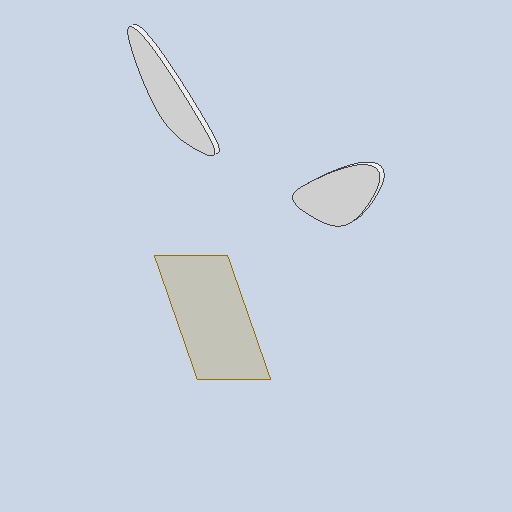
# Autodesk Inventor part: втавки в уши
Saved by Autodesk Inventor 2024.2 (Build 282272000, 272)
## iProperties
Created: 2026-04-13
Part Number: втавки в уши
Material: Типовые
Document SubType Name: Modeling
Designer: katya_notebook
Density: 1 g/cm^3
Appearance: Белый
Author: katya_notebook
Autodesk Inventor part; units mm, degrees
ref_plane "YZ Plane" through (0, 0, 0) normal (1, 0, 0) x (0, 1, 0)
ref_plane "XZ Plane" through (0, 0, 0) normal (0, 1, 0) x (-1, 0, 0)
ref_plane "XY Plane" through (0, 0, 0) normal (0, 0, 1) x (1, 0, 0)
ref_plane "РабПлоскость1" through (35.0491, -167.4778, 0) normal (0, 0, 1) x (-0.4483757, 0.8938452, 0)
sketch "Эскиз1" plane through (35.0491, -167.4778, 0) normal (0, 0, 1) x (-0.4483757, 0.8938452, 0)
  spline S0 degree 3 poles (119.1304, -59.9769) (121.6559, -53.204) (124.3274, -47.3227) (129.9976, -38.042) (132.8145, -34.5593) (139.864, -28.2576) (144.2541, -25.75) (161.0383, -19.7449) (176.2169, -18.9451) (191.3353, -18.7692) (197.9842, -18.9943) (204.6873, -20.2717) (206.5014, -20.7653) (208.7394, -21.856) (209.4736, -22.3119) (210.4771, -23.27) (210.8203, -23.7079) (211.3082, -24.6937) (211.4431, -25.2098) (211.5165, -26.4335) (211.3928, -27.1121) (210.789, -28.8946) (210.0931, -29.9834) (207.1495, -33.7221) (203.6117, -36.415) (190.7312, -44.8629) (177.0786, -50.9399) (157.9772, -58.7745) (140.9066, -65.3521) (129.32, -68.3562) (126.8697, -68.8535) (123.8804, -68.9432) (122.9917, -68.8784) (121.6982, -68.5374) (121.2096, -68.337) (120.3608, -67.7605) (120.0208, -67.412) (119.3919, -66.448) (119.1764, -65.822) (118.7753, -63.8427) (118.8182, -62.121) (119.1304, -59.9769) knots -19.535718 -19.535718 -19.535718 -19.535718 -18.521729 -18.521729 -17.645169 -17.645169 -16.585337 -16.585337 -14.272905 -14.272905 -12.64955 -12.64955 -12.036111 -12.036111 -11.729258 -11.729258 -11.523538 -11.523538 -11.322846 -11.322846 -11.070518 -11.070518 -10.627583 -10.627583 -9.313537 -9.313537 -5.689602 -5.689602 -2.653594 -2.653594 -1.828822 -1.828822 -1.444244 -1.444244 -1.194814 -1.194814 -0.958616 -0.958616 -0.650005 -0.650005 0 0 0 0 projected
  spline S1 degree 3 poles (81.1608, -135.4055) (82.6694, -133.905) (84.0051, -132.8572) (85.7594, -132.0121) (86.3344, -131.8139) (87.4209, -131.6843) (87.9054, -131.7157) (88.9368, -132.0027) (89.437, -132.2802) (90.5464, -133.1347) (91.1457, -133.8196) (92.6734, -135.997) (93.6462, -137.8968) (98.3538, -149.2241) (103.4784, -167.8703) (108.7593, -188.6993) (111.9298, -203.3921) (112.5266, -217.9445) (112.4209, -221.5049) (111.474, -225.6569) (111.0615, -226.9332) (110.0933, -228.6044) (109.6715, -229.1618) (108.7472, -229.9574) (108.2942, -230.2289) (107.2526, -230.589) (106.6952, -230.6521) (105.309, -230.5683) (104.4974, -230.3167) (102.2449, -229.3087) (100.7345, -228.1844) (96.8673, -224.7585) (93.9765, -221.509) (86.2996, -211.6092) (78.659, -200.9063) (70.8126, -183.9525) (69.4544, -179.1485) (68.0007, -169.9558) (68.2614, -164.9864) (71.2214, -152.8149) (74.9276, -145.0071) (81.1608, -135.4055) knots -41.696489 -41.696489 -41.696489 -41.696489 -40.089473 -40.089473 -39.380109 -39.380109 -38.790822 -38.790822 -38.109795 -38.109795 -37.126857 -37.126857 -35.423768 -35.423768 -29.350664 -29.350664 -21.057196 -21.057196 -18.450357 -18.450357 -17.370914 -17.370914 -16.777508 -16.777508 -16.314434 -16.314434 -15.822726 -15.822726 -15.111611 -15.111611 -13.684583 -13.684583 -11.140705 -11.140705 -7.811331 -7.811331 -5.919376 -5.919376 -3.434235 -3.434235 0 0 0 0 projected
  point P0 (165.4144, -43.7645)
  point P1 (119.1304, -59.9769)
  point P2 (81.1608, -135.4055)
extrude "Выдавливание1" add sketch "Эскиз1" along normal blind 4
